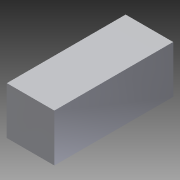
# Autodesk Inventor part: container
Saved by Autodesk Inventor 2014 SP1 (Build 180222100, 222)
## iProperties
Created: 2014-02-26
Part Number: container
Material: UHMW, White
Document SubType Name: Modeling
Designer: Dave
Mass: 3.24864e+07 g
Surface Area: 691200 cm^2
Volume: 3.456e+07 cm^3
Density: 0.94 g/cm^3
Appearance: Smooth - White
Author: Dave
Autodesk Inventor part; units mm, degrees
ref_plane "YZ Plane" through (0, 0, 0) normal (1, 0, 0) x (0, 1, 0)
ref_plane "XZ Plane" through (0, 0, 0) normal (0, 1, 0) x (-1, 0, 0)
ref_plane "XY Plane" through (0, 0, 0) normal (0, 0, 1) x (1, 0, 0)
sketch "Sketch1" plane through (0, 0, 0) normal (0, 1, 0) x (-1, 0, 0)
  line L0 (0, 0) -> (-2400, 0)
  line L1 (-2400, 0) -> (-2400, -6000)
  line L2 (-2400, -6000) -> (0, -6000)
  line L3 (0, -6000) -> (0, 0)
  dimension "d0" = 2400
  dimension "d1" = 6000
  constraints: 8 end point, 2 parallel, 1 horizontal, 1 perpendicular
  measures "d0" distance of L0.start L0.end
  measures "d1" distance of L2.end L0.start
extrude "Extrusion1" add sketch "Sketch1" along normal blind 2400
body "Solid1"
